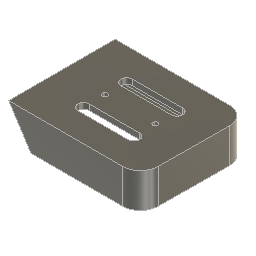
Крепление аккамулятора Milwaukee_ver2 (Autodesk Fusion 360 design; units mm, degrees)
Autodesk Fusion 360 part; units mm, degrees
note: some values were not read from the file. Set by a fixed rule: which sketch regions a step uses.
sketch "Sketch1" plane through (0, 0, 0) normal (0, 0, 1) x (1, 0, 0)
  line L0 (34.5, 30.5) -> (-32.5, 30.5)
  line L1 (-32.5, 30.5) -> (-32.5, -30.5)
  line L2 (-32.5, -30.5) -> (34.5, -30.5)
  line L3 (34.5, -30.5) -> (34.5, 30.5)
  line L4 (34.5, -27.25) -> (-32.5, -27.25)
  line L5 (-32.5, -27.25) -> (-32.5, 27.25)
  line L6 (-32.5, 27.25) -> (34.5, 27.25)
  line L7 (34.5, 27.25) -> (34.5, -27.25)
  line L8 (29.4153, 37) -> (-32.5, 37)
  line L9 (-32.5, 37) -> (-32.5, 30.5)
  line L10 (1.75, 0) -> (22.5, 0)
  line L11 (-32.5, -37) -> (-32.5, -30.5)
  line L12 (29.0842, -37) -> (-32.5, -37)
  line L13 (41.5839, -24.5845) -> (41.915, 24.4155)
  arc A0 (41.915, 24.4155) -> (29.4153, 37) centre (29.4153, 24.5) ccw
  arc A1 (29.0842, -37) -> (41.5839, -24.5845) centre (29.0842, -24.5) ccw
  dimension "d1" = 67
  dimension "d2" = 61
  dimension "d3" = 67
  dimension "d4" = 54.5
  dimension "d32" = 12.5
  constraint horizontal L0
  constraint perpendicular L0 L1
  constraint parallel L0 L2
  constraint parallel L1 L3
  constraint horizontal L4
  constraint perpendicular L4 L5
  constraint parallel L4 L6
  constraint parallel L5 L7
  constraint perpendicular L0 L9
  constraint symmetric L0.end L10 L1.end
  constraint symmetric L8.end L10 L11.start
  constraint tangent L8 A0
  constraint tangent L13 A0
  constraint tangent L12 A1
  constraint tangent L13 A1
  constraint equal A0 A1
  measures "d1" distance of L1.end L2.end
  measures "d2" distance of L0.end L1.end
  measures "d3" distance of L5.end L6.end
  measures "d4" distance of L4.end L5.end
  measures "d32" radius of A0
extrude "Extrude1" add sketch "Sketch1" along normal blind 6.6 contours L0 L1 L3 L6 | L0 L2 L3 L7 L8 L9 L11 L12 L13 A0 A1 | L1 L2 L3 L4
extrude "Extrude2" add sketch "Sketch1" along normal blind 22 contours L0 L2 L3 L7 L8 L9 L11 L12 L13 A0 A1
extrude "Extrude3" add sketch "Sketch1" along normal blind 24 and the other way blind -20
sketch "Sketch2" plane through (0, 0, 24) normal (0, 0, 1) x (-1, 0, 0)
  line L0 (-29.4153, -37) -> (32.5, -37)
  line L1 (32.5, -37) -> (32.5, 37)
  line L2 (32.5, 37) -> (-29.0842, 37)
  line L3 (-41.5839, 24.5845) -> (-41.915, -24.4155)
  arc A0 (-29.0842, 37) -> (-41.5839, 24.5845) centre (-29.0842, 24.5) ccw
  arc A1 (-41.915, -24.4155) -> (-29.4153, -37) centre (-29.4153, -24.5) ccw
  circle A2 centre (20, 0) radius 1.75
  circle A3 centre (-15, 0) radius 1.75
  dimension "d33" = 3.5
  dimension "d34" = 3.5
  measures "d33" diameter of A2
  measures "d34" diameter of A3
extrude "Extrude4" cut sketch "Sketch2" against normal blind 5 contours A2 | A3
sketch "Sketch3" plane through (0, 37, 0) normal (0, 1, 0) x (-1, 0, 0)
  line L0 (-29.4153, 0) -> (32.5, 0)
  line L1 (32.5, 0) -> (32.5, 24)
  line L2 (32.5, 24) -> (-29.4153, 24)
  line L3 (32.5, 24) -> (34.5, 24)
  line L4 (34.5, 24) -> (34.5, 0)
  line L5 (34.5, 0) -> (32.5, 0)
  line L6 (34.5, 0) -> (34.5, 8)
  line L7 (-29.4153, 24) -> (-29.4153, 0)
  line L8 (34.5, 24) -> (50.0216, 24)
  line L9 (34.5, 0) -> (50.0216, 24)
  constraint coincident L1.end L2.start
  constraint perpendicular L1 L3
  constraint perpendicular L3 L4
  constraint coincident L0.end L1.start
  constraint perpendicular L1 L5
  constraint coincident L4 L6.end
  constraint perpendicular L4 L8
extrude "Extrude5" add sketch "Sketch3" against normal blind 6.5 contours L1 L3 L4 L5 L6 | L4 L6 L8 L9
extrude "Extrude6" add sketch "Sketch3" along normal blind -74 and the other way blind 67.5 contours L1 L3 L4 L5 L6 | L4 L6 L8 L9
sketch "Sketch4" plane through (0, 30.5, 0) normal (0, -1, 0) x (1, 0, 0)
  line L0 (-32.5, 6.6) -> (34.5, 6.6)
  line L1 (34.5, 6.6) -> (34.5, 20)
  line L2 (34.5, 20) -> (-32.5, 20)
  line L3 (-32.5, 20) -> (-32.5, 24)
  line L4 (-32.5, 24) -> (-50.0216, 24)
  line L5 (-50.0216, 24) -> (-34.5, 0)
  line L6 (-34.5, 0) -> (-38.7684, 6.6)
  line L7 (-32.5, 6.6) -> (-38.7684, 6.6)
  line L8 (-32.5, 6.6) -> (-32.5, 0)
  line L9 (-34.5, 0) -> (-32.5, 0)
  constraint coincident L5.end L6.start
  constraint coincident L0.start L7.start
  constraint parallel L0 L7
  constraint perpendicular L7 L8
  constraint perpendicular L8 L9
  constraint coincident L5 L6.end
extrude "Extrude7" add sketch "Sketch4" along normal blind 3.25 contours L5 L6 L7 L8 L9
extrude "Extrude8" add sketch "Sketch4" along normal blind 61 and the other way blind -57.75 contours L5 L6 L7 L8 L9
chamfer "Chamfer2" distance 1 angle 45 2 edges at (-18.3684, 0.6328, 20) (16.6316, 0.6328, 20)
sketch "Sketch5" plane through (0, 30.5, 0) normal (0, -1, 0) x (1, 0, 0)
  line L0 (-38.7684, 6.6) -> (34.5, 6.6)
  line L1 (34.5, 6.6) -> (34.5, 20)
  line L2 (34.5, 20) -> (-32.5, 20)
  line L3 (-32.5, 20) -> (-32.5, 24)
  line L4 (-32.5, 24) -> (-50.0216, 24)
  line L5 (-50.0216, 24) -> (-38.7684, 6.6)
  line L6 (-50.0216, 24) -> (-32.5, 24)
  line L7 (-32.5, 20) -> (-47.4346, 20)
  line L8 (-50.0216, 24) -> (-47.4346, 20)
  constraint coincident L4.end L5.start
  constraint coincident L3.end L4.start
  constraint coincident L2.end L3.start
  constraint perpendicular L3 L7
  constraint coincident L5 L7.end
extrude "Extrude9" add sketch "Sketch5" along normal blind 61 contours L3 L4 L5 L6 L7 L8
sketch "Sketch6" plane through (0, 0, 20) normal (0, 0, -1) x (1, 0, 0)
  circle A0 centre (-20, 0) radius 2.75
  line L0 (34.5, 30.5) -> (-47.4346, 30.5)
  line L1 (-47.4346, 30.5) -> (-47.4346, -30.5)
  line L2 (-47.4346, -30.5) -> (34.5, -30.5)
  line L3 (34.5, -30.5) -> (34.5, 30.5)
  circle A1 centre (15, 0) radius 2.75
  line L4 (15, -11) -> (-20, -11)
  arc A2 (-20, -11) -> (-20, -19) centre (-20, -15) ccw
  line L5 (-20, -19) -> (15, -19)
  arc A3 (15, -19) -> (15, -11) centre (15, -15) ccw
  line L6 (15, -15) -> (-20, -15) construction
  line L7 (1.75, 0) -> (22.5, 0)
  line L8 (-20, 19) -> (15, 19)
  arc A4 (15, 11) -> (15, 19) centre (15, 15) ccw
  line L9 (15, 11) -> (-20, 11)
  arc A5 (-20, 19) -> (-20, 11) centre (-20, 15) ccw
  constraint tangent L4 A2
  constraint tangent A2 L5
  constraint parallel L4 L5
  constraint tangent L5 A3
  constraint tangent L4 A3
  constraint horizontal L6
  constraint symmetric L4.start L7 A4.start
  constraint symmetric L4.end L7 L9.end
  constraint symmetric A2.end L7 L8.start
  constraint symmetric L5.end L7 L8.end
  constraint symmetric A2 L7 A5
  constraint symmetric A3 L7 A4
extrude "Extrude10" cut sketch "Sketch6" against normal blind 25 contours L4 A2 L5 A3 | L8 A4 L9 A5
